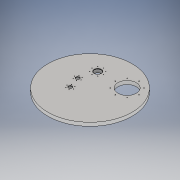
# Autodesk Inventor part: Top Plate
Saved by Autodesk Inventor 2018 (Build 220112000, 112)
## iProperties
Created: 2018-08-07
Part Number: Top Plate
Material: Generic
Document SubType Name: Modeling
Designer: freyja
Density: 1 g/cm^3
Appearance: Default
Author: freyja
Autodesk Inventor part; units mm, degrees
ref_plane "YZ Plane" through (0, 0, 0) normal (1, 0, 0) x (0, 1, 0)
ref_plane "XZ Plane" through (0, 0, 0) normal (0, 1, 0) x (-1, 0, 0)
ref_plane "XY Plane" through (0, 0, 0) normal (0, 0, 1) x (1, 0, 0)
sketch "Sketch1" plane through (0, 0, 0) normal (0, 1, 0) x (-1, 0, 0)
  line L0 (609.6, 609.6) -> (-609.6, 609.6)
  line L1 (-609.6, 609.6) -> (-609.6, -609.6)
  line L2 (-609.6, -609.6) -> (609.6, -609.6)
  line L3 (609.6, -609.6) -> (609.6, 609.6)
  line L4 (609.6, 609.6) -> (-609.6, -609.6) construction
  line L5 (-609.6, 609.6) -> (609.6, -609.6) construction
  point P0 (0, 0)
  dimension "d0" = 1219.2
  dimension "d1" = 1219.2
  constraints: 12 end point, 2 midpoint, 2 parallel, 1 horizontal, 1 perpendicular
  measures "d0" distance of L2.end L1.end
  measures "d1" distance of L1.end L0.end
extrude "Extrusion1" add sketch "Sketch1" along normal blind 25.4
sketch "Sketch2" plane through (0, 25.4, 0) normal (0, 1, 0) x (1, 0, 0)
  line L0 (0, 0) -> (134.7038, 134.7038) construction
  line L1 (0, 0) -> (190.5, 0) construction
  circle A0 centre (134.7038, 134.7038) radius 118.745 construction
  circle A1 centre (134.7038, 134.7038) radius 66.675
  dimension "d4" = 190.5
  dimension "d5" = 45
  dimension "d6" = 237.49
  dimension "d7" = 133.35
  constraints: 4 end point, 2 centre point, 2 coincident, 1 equal length, 1 horizontal
  measures "d4" distance of L0.start L0.end
  measures "d5" angle of L1 L0
  measures "d6" diameter of A0
  measures "d7" diameter of A1
extrude "Extrusion2" cut sketch "Sketch2" against normal up to surface (25.4 mm away)
sketch "Sketch10" plane through (0, 25.4, 0) normal (0, 1, 0) x (1, 0, 0)
  circle A0 centre (0, 0) radius 304.8
  dimension "d65" = 609.6
  constraints: 1 centre point, 1 coincident
  measures "d65" diameter of A0
extrude "Extrusion7" cut sketch "Sketch10" against normal up to surface (25.4 mm away) keep common part
sketch "Sketch3" plane through (0, 25.4, 0) normal (0, 1, 0) x (1, 0, 0)
  circle A0 centre (134.7038, 134.7038) radius 66.675 projected
  line L0 (134.7038, 134.7038) -> (221.0638, 134.7038) construction
  line L1 (134.7038, 134.7038) -> (221.0638, 134.7038) construction
  line L2 (134.7038, 134.7038) -> (195.7696, 195.7696) construction
  line L3 (134.7038, 134.7038) -> (134.7038, 221.0638) construction
  line L4 (134.7038, 134.7038) -> (73.6381, 195.7696) construction
  line L5 (134.7038, 134.7038) -> (48.3438, 134.7038) construction
  line L6 (134.7038, 134.7038) -> (73.6381, 73.6381) construction
  line L7 (134.7038, 134.7038) -> (134.7038, 48.3438) construction
  line L8 (134.7038, 134.7038) -> (195.7696, 73.6381) construction
  point P0 (0, 0)
  dimension "d10" = 86.36
  dimension "d11" = 0
  dimension "d14" = 360
  constraints: 18 end point, 2 coincident, 2 horizontal, 1 collinear, 23 other
  measures "d10" distance of L0.start L0.end
  measures "d11" distance between parallel lines of L0 L1
hole "Hole1" at (221.0638, 25.4, -134.7038) at (195.7696, 25.4, -195.7696) at (134.7038, 25.4, -221.0638) at (73.6381, 25.4, -195.7696) at (48.3438, 25.4, -134.7038) at (73.6381, 25.4, -73.6381) at (134.7038, 25.4, -48.3438) at (195.7696, 25.4, -73.6381) direction (0, -1, 0) diameter 4.9784 depth 19.05 tip angle 118 thread size "1/4-20 UNC" class "2B" standard "ANSI Unified Screw Threads"
sketch "Sketch4" plane through (0, 25.4, 0) normal (0, 1, 0) x (1, 0, 0)
  line L0 (0, 0) -> (-76.2, 131.9823) construction
  line L1 (0, 0) -> (152.4, 0) construction
  circle A0 centre (-76.2, 131.9823) radius 26.289
  dimension "d23" = 152.4
  dimension "d24" = 120
  dimension "d25" = 52.578
  constraints: 4 end point, 1 centre point, 1 coincident, 1 equal length, 1 horizontal
  measures "d23" distance of L0.start L0.end
  measures "d24" angle of L1 L0
  measures "d25" diameter of A0
extrude "Extrusion3" cut sketch "Sketch4" against normal blind 2.54
sketch "Sketch5" plane through (-76.2, 22.86, -131.9823) normal (0, 1, 0) x (1, 0, 0)
  circle A0 centre (0, 0) radius 26.289 projected
  circle A1 centre (0, 0) radius 24.13
  point P0 (76.2, -131.9823)
  dimension "d28" = 48.26
  constraints: 1 centre point, 1 coincident
  measures "d28" diameter of A1
extrude "Extrusion4" cut sketch "Sketch5" against normal up to surface (22.86 mm away) contours A1
sketch "Sketch6" plane through (0, 25.4, 0) normal (0, 1, 0) x (1, 0, 0)
  circle A0 centre (-76.2, 131.9823) radius 24.13 construction
  line L0 (-76.2, 131.9823) -> (-34.925, 131.9823) construction
  line L1 (-76.2, 131.9823) -> (-34.925, 131.9823) construction
  line L2 (-76.2, 131.9823) -> (-47.0142, 161.1681) construction
  line L3 (-76.2, 131.9823) -> (-76.2, 173.2573) construction
  line L4 (-76.2, 131.9823) -> (-105.3858, 161.1681) construction
  line L5 (-76.2, 131.9823) -> (-117.475, 131.9823) construction
  line L6 (-76.2, 131.9823) -> (-105.3858, 102.7964) construction
  line L7 (-76.2, 131.9823) -> (-76.2, 90.7073) construction
  line L8 (-76.2, 131.9823) -> (-47.0142, 102.7964) construction
  point P0 (0, 0)
  dimension "d31" = 41.275
  dimension "d32" = 0
  dimension "d35" = 360
  constraints: 18 end point, 2 coincident, 2 horizontal, 1 collinear, 23 other
  measures "d31" distance of L0.start L0.end
  measures "d32" distance between parallel lines of L0 L1
hole "Hole2" at (-47.0142, 25.4, -161.1681) at (-76.2, 25.4, -173.2573) at (-105.3858, 25.4, -161.1681) at (-117.475, 25.4, -131.9823) at (-105.3858, 25.4, -102.7964) at (-76.2, 25.4, -90.7073) at (-47.0142, 25.4, -102.7964) at (-34.925, 25.4, -131.9823) direction (0, -1, 0) diameter 3.9624 depth 13.6144 tip angle 118 thread size "10-32 UNF" class "2B" standard "ANSI Unified Screw Threads"
sketch "Sketch7" plane through (0, 25.4, 0) normal (0, 1, 0) x (1, 0, 0)
  line L0 (0, 0) -> (-77.8301, -65.3072) construction
  line L1 (0, 0) -> (101.6, 0) construction
  circle A0 centre (-77.8301, -65.3072) radius 13.208
  dimension "d44" = 101.6
  dimension "d45" = 220
  dimension "d46" = 26.416
  constraints: 4 end point, 1 centre point, 1 coincident, 1 equal length, 1 horizontal
  measures "d44" distance of L0.start L0.end
  measures "d46" diameter of A0
extrude "Extrusion5" cut sketch "Sketch7" against normal blind 2.54
sketch "Sketch8" plane through (0, 25.4, 0) normal (0, 1, 0) x (1, 0, 0)
  circle A0 centre (-77.8301, -65.3072) radius 13.208 projected
  circle A1 centre (-77.8301, -65.3072) radius 11.43
  point P0 (0, 0)
  dimension "d49" = 22.86
  constraints: 1 centre point, 1 coincident
  measures "d49" diameter of A1
extrude "Extrusion6" cut sketch "Sketch8" against normal up to surface (25.4 mm away) contours A1
sketch "Sketch9" plane through (0, 25.4, 0) normal (0, 1, 0) x (1, 0, 0)
  circle A0 centre (-77.8301, -65.3072) radius 13.208 projected
  line L0 (-77.8301, -65.3072) -> (-53.8271, -65.3072) construction
  line L1 (-77.8301, -65.3072) -> (-53.8271, -65.3072) construction
  line L2 (-77.8301, -65.3072) -> (-65.8286, -44.52) construction
  line L3 (-77.8301, -65.3072) -> (-89.8316, -44.52) construction
  line L4 (-77.8301, -65.3072) -> (-101.8331, -65.3072) construction
  line L5 (-77.8301, -65.3072) -> (-89.8316, -86.0944) construction
  line L6 (-77.8301, -65.3072) -> (-65.8286, -86.0944) construction
  point P0 (0, 0)
  dimension "d52" = 24.003
  dimension "d53" = 0
  dimension "d56" = 360
  constraints: 14 end point, 2 coincident, 2 horizontal, 1 collinear, 17 other
  measures "d52" distance of L0.start L0.end
  measures "d53" distance between parallel lines of L0 L1
hole "Hole3" at (-53.8271, 25.4, 65.3072) at (-65.8286, 25.4, 44.52) at (-89.8316, 25.4, 44.52) at (-101.8331, 25.4, 65.3072) at (-89.8316, 25.4, 86.0944) at (-65.8286, 25.4, 86.0944) direction (0, -1, 0) diameter 3.9624 depth 13.6144 tip angle 118 thread size "10-32 UNF" class "2B" standard "ANSI Unified Screw Threads"
sketch "Sketch11" plane through (-11.3966, 25.4, -31.3943) normal (0, 1, 0) x (1, 0, 0)
  line L0 (6.079, -13.3722) -> (-95.521, -13.3722) construction
  line L1 (6.079, -13.3722) -> (107.679, -13.3722) construction
  circle A0 centre (-95.521, -13.3722) radius 13.208
  dimension "d70" = 101.6
  dimension "d69" = 180
  dimension "d68" = 26.416
  constraints: 4 end point, 1 centre point, 1 coincident, 1 collinear, 1 horizontal
  measures "d70" distance of L0.start L0.end
  measures "d69" angle of L1 L0
  measures "d68" diameter of A0
extrude "Extrusion8" cut sketch "Sketch11" against normal blind 2.54
sketch "Sketch12" plane through (0, 25.4, 0) normal (0, 1, 0) x (-1, 0, 0)
  circle A0 centre (106.9176, -18.0221) radius 13.208 projected
  circle A1 centre (106.9176, -18.0221) radius 11.43
  point P0 (0, 0)
  dimension "d74" = 22.86
  constraints: 1 centre point, 1 coincident
  measures "d74" diameter of A1
extrude "Extrusion9" cut sketch "Sketch12" against normal up to surface (25.4 mm away) contours A1
sketch "Sketch13" plane through (0, 25.4, 0) normal (0, 1, 0) x (-1, 0, 0)
  circle A0 centre (106.9176, -18.0221) radius 13.208 projected
  line L0 (106.9176, -18.0221) -> (130.9206, -18.0221) construction
  line L1 (106.9176, -18.0221) -> (130.9206, -18.0221) construction
  line L2 (106.9176, -18.0221) -> (118.9191, 2.7651) construction
  line L3 (106.9176, -18.0221) -> (94.9161, 2.7651) construction
  line L4 (106.9176, -18.0221) -> (82.9146, -18.0221) construction
  line L5 (106.9176, -18.0221) -> (94.9161, -38.8093) construction
  line L6 (106.9176, -18.0221) -> (118.9191, -38.8093) construction
  point P0 (0, 0)
  dimension "d82" = 24.003
  dimension "d89" = 0
  dimension "d81" = 360
  constraints: 14 end point, 2 coincident, 2 horizontal, 1 collinear, 17 other
  measures "d82" distance of L0.start L0.end
  measures "d89" distance between parallel lines of L0 L1
hole "Hole4" at (-130.9206, 25.4, -18.0221) at (-118.9191, 25.4, 2.7651) at (-94.9161, 25.4, 2.7651) at (-82.9146, 25.4, -18.0221) at (-94.9161, 25.4, -38.8093) at (-118.9191, 25.4, -38.8093) direction (0, -1, 0) diameter 3.9624 depth 13.6144 tip angle 118
body "Solid1"
